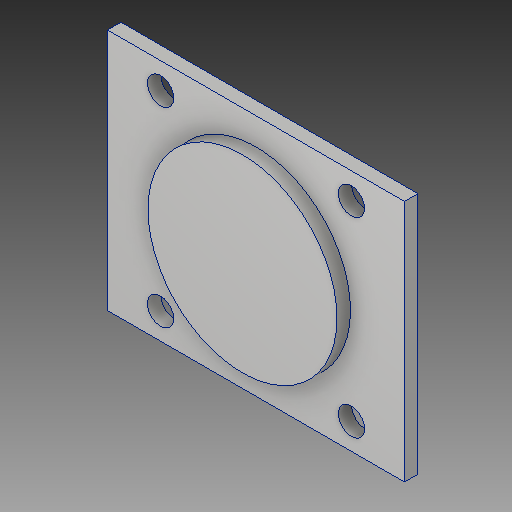
# Autodesk Inventor part: endcap1
Saved by Autodesk Inventor 2018.1 (Build 221171000, 171)
## iProperties
Created: 2017-09-01
Part Number: endcap1
Material: Aluminum 6061
Document SubType Name: Modeling
Designer: Kai
Density: 2.7 g/cm^3
Appearance: Aluminum - Flat
Author: Kai
Autodesk Inventor part; units mm, degrees
ref_plane "YZ Plane" through (0, 0, 0) normal (1, 0, 0) x (0, 1, 0)
ref_plane "XZ Plane" through (0, 0, 0) normal (0, 1, 0) x (-1, 0, 0)
ref_plane "XY Plane" through (0, 0, 0) normal (0, 0, 1) x (1, 0, 0)
sketch "Sketch1" plane through (0, 0, 0) normal (0, 0, 1) x (1, 0, 0)
  line L0 (0, 0) -> (-69.85, 0)
  line L1 (-69.85, 0) -> (-69.85, 57.15)
  line L2 (-69.85, 57.15) -> (0, 57.15)
  line L3 (0, 57.15) -> (0, 0)
  dimension "d0" = 69.85
  dimension "d1" = 57.15
  constraints: 8 end point, 2 parallel, 1 horizontal, 1 perpendicular
  measures "d0" distance of L1.end L2.end
  measures "d1" distance of L0.end L1.end
extrude "Extrusion1" add sketch "Sketch1" along normal blind 3.175
sketch "Sketch2" plane through (0, 0, 3.175) normal (0, 0, 1) x (1, 0, 0)
  line L0 (-69.85, 57.15) -> (-69.85, 0) construction
  line L1 (-69.85, 0) -> (0, 0) construction
  line L2 (-69.85, 57.15) -> (0, 0) construction
  circle A0 centre (-34.925, 28.575) radius 22.225
  dimension "d4" = 44.45
  constraints: 2 end point, 1 centre point, 1 midpoint
  measures "d4" diameter of A0
extrude "Extrusion2" add sketch "Sketch2" along normal blind 3.175
sketch "Sketch3" plane through (0, 0, 3.175) normal (0, 0, 1) x (1, 0, 0)
  circle A0 centre (-34.925, 28.575) radius 22.225 construction
  circle A1 centre (-34.925, 28.575) radius 31.75 construction
  line L0 (-34.925, 28.575) -> (-12.4744, 6.1244) construction
  line L1 (-34.925, 28.575) -> (-3.175, 28.575) construction
  circle A2 centre (-12.4744, 6.1244) radius 3.1
  circle A3 centre (-12.4744, 51.0256) radius 3.1
  circle A4 centre (-57.3756, 51.0256) radius 3.1
  circle A5 centre (-57.3756, 6.1244) radius 3.1
  point P0 (0, 0)
  dimension "d7" = 63.5
  dimension "d8" = 45
  dimension "d9" = 6.2
  dimension "d12" = 360
  constraints: 4 centre point, 4 end point, 2 coincident, 1 equal length, 1 horizontal, 12 other
  measures "d8" angle of L0 L1
  measures "d9" diameter of A2
extrude "Extrusion3" cut sketch "Sketch3" against normal blind 3.175
body "Solid1"
